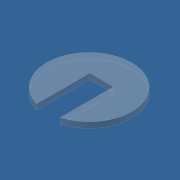
# Autodesk Inventor part: S1702_couverclerailressort
Saved by Autodesk Inventor 2015 SP2 (Build 190223200, 223)
## iProperties
Created: 2017-10-31
Part Number: S1702_couverclerailressort
Project: S1701_Circuit_Course_Manette
Material: Plastique PMMA
Description: Plaque Rail Ressort
Document SubType Name: Modeling
Designer: Benoit.CURCHOD2
Authority: Ø44x3
Density: 1.188 g/cm^3
Appearance: Transparent - Clair
Mass: 3.43675 g
Surface Area: 30.326 cm^2
Volume: 2.89288 cm^3
Material number: ---
Author: Benoit.CURCHOD2
Autodesk Inventor part; units mm, degrees
ref_plane "Plan YZ" through (0, 0, 0) normal (1, 0, 0) x (0, 1, 0)
ref_plane "Plan XZ" through (0, 0, 0) normal (0, 1, 0) x (-1, 0, 0)
ref_plane "Plan XY" through (0, 0, 0) normal (0, 0, 1) x (1, 0, 0)
sketch "Esquisse1" plane through (0, 0, 0) normal (0, 0, 1) x (1, 0, 0)
  arc A0 (6.15, -21.1229) -> (-6.15, -21.1229) centre (0, 0) ccw
  line L0 (-6.15, 6.5) -> (6.15, 6.5)
  line L1 (6.15, 6.5) -> (6.15, -21.1229)
  line L2 (-6.15, -21.1229) -> (-6.15, 6.5)
  line L3 (-30.8, 0) -> (30.8, 0) construction
  line L4 (0, -29.7475) -> (0, 30.6246) construction
  circle A1 centre (-12.5, 14.0424) radius 1.7
  circle A2 centre (12.5, 14.0424) radius 1.7
  circle A3 centre (10, -15.9198) radius 1.7
  circle A4 centre (-10, -15.9198) radius 1.7
  circle A5 centre (0, 0) radius 18.8 construction
  dimension "d0" = 44
  dimension "d2" = 12.3
  dimension "d43" = 6.5
  dimension "d44" = 3.4
  dimension "d45" = 25
  dimension "d46" = 20
  dimension "d47" = 37.6
  constraints: 6 centre point, 6 end point, 6 point on circle, 1 coincident, 1 equal radius, 1 horizontal, 1 parallel, 1 perpendicular, 3 other
  measures "d0" diameter of A0
  measures "d2" distance of L0.start L0.end
  measures "d43" distance between parallel lines of L3 L0
  measures "d44" diameter of A1
  measures "d45" distance of A1.centre A2.centre
  measures "d46" distance of A3.centre A4.centre
  measures "d47" diameter of A5
extrude "Extrusion1" add sketch "Esquisse1" along normal blind 3 contours L1 L0 L2 A0 | A1 | A2 | A3 | A4
sketch "Esquisse7" plane through (0, 0, 3) normal (0, 0, 1) x (1, 0, 0)
  circle A0 centre (-12.5, 14.0424) radius 1.7
  line L0 (0, -29.7475) -> (0, 30.6246) construction
  circle A1 centre (12.5, 14.0424) radius 1.7
  circle A2 centre (10, -15.9198) radius 1.7
  line L1 (-30.8, 0) -> (30.8, 0) construction
  circle A3 centre (-10, -15.9198) radius 1.7
  circle A4 centre (0, 0) radius 18.8 construction
  dimension "d23" = 3.4
  dimension "d33" = 25
  dimension "d34" = 20
  dimension "d42" = 37.6
  constraints: 5 centre point, 2 point on circle, 2 symmetric about line, 1 coincident, 1 equal radius, 2 other
  measures "d23" diameter of A0
  measures "d33" distance of A0.centre A1.centre
  measures "d34" distance of A2.centre A3.centre
  measures "d42" diameter of A4
sketch "Esquisse8" plane through (0, 0, 0) normal (0, 0, -1) x (-1, 0, 0)
  line L0 (30.8, 0) -> (-30.8, 0) construction
  line L1 (0, -29.7475) -> (0, 30.6246) construction
  line L2 (-12.5, -10) -> (12.5, -10) construction
  line L3 (12.5, -10) -> (12.5, -11.7) construction
  line L4 (12.5, -11.7) -> (-12.5, -11.7) construction
  line L5 (-12.5, -11.7) -> (-12.5, -10) construction
  line L6 (-6.15, 6.5) -> (-6.15, -21.1229) construction
  line L7 (6.15, -21.1229) -> (6.15, 6.5) construction
  line L8 (-6.15, -10) -> (-12.5, -10)
  line L9 (-12.5, -11.7) -> (-12.5, -10)
  line L10 (-6.15, -11.7) -> (-6.15, -10)
  line L11 (-6.15, -11.7) -> (-12.5, -11.7)
  line L12 (6.15, -11.7) -> (6.15, -10)
  line L13 (6.15, -21.1229) -> (6.15, 6.5) projected
  line L14 (6.15, -10) -> (12.5, -10)
  line L15 (12.5, -10) -> (12.5, -11.7)
  line L16 (12.5, -11.7) -> (6.15, -11.7)
  point P0 (0, 0)
  dimension "d28" = 1.7
  dimension "d29" = 25
  dimension "d30" = 10
  constraints: 24 end point, 8 point on line, 7 collinear, 2 parallel, 1 horizontal, 1 perpendicular, 1 other
  measures "d28" distance between parallel lines of L2 L4
  measures "d29" distance between parallel lines of L3 L5
  measures "d30" distance between parallel lines of L2 L0
